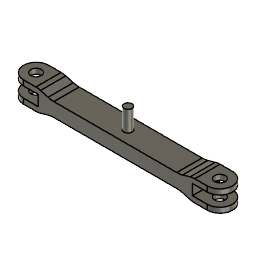
BARRA_SERVO (Autodesk Fusion 360 design; units mm, degrees)
Autodesk Fusion 360 part; units mm, degrees
sketch "Boceto1" plane through (0, 0, 0) normal (0, 0, 1) x (1, 0, 0)
  line L0 (-43.4775, 6) -> (43.4775, 6)
  circle A0 centre (0, 0) radius 1.95
  line L1 (-36.4775, 6) -> (-36.4775, -6)
  line L2 (36.4775, 6) -> (36.4775, -6)
  line L3 (-30.4775, 6) -> (-30.4775, -6)
  line L4 (30.4775, 6) -> (30.4775, -6)
  circle A1 centre (-43.4775, 0) radius 2 construction
  circle A2 centre (43.4775, 0) radius 2 construction
  line L5 (-43.4775, 0) -> (43.4775, 0) construction
  line L6 (-43.4868, -6) -> (43.4868, -6)
  arc A3 (-43.4775, 6) -> (-43.4868, -6) centre (-43.4775, 0) ccw
  arc A4 (43.4868, -6) -> (43.4775, 6) centre (43.4775, 0) ccw
  circle A5 centre (-43.4775, 0) radius 2.5
  circle A6 centre (43.4775, 0) radius 2.5
  line L7 (57, 0) -> (-57, 0) construction
  line L8 (0, -7.1894) -> (0, 7.1894) construction
  point P0 (0, -6)
  point P1 (0, 6)
  dimension "d8" = 3.9
  dimension "d9" = 86.955
  dimension "d16" = 6
  dimension "d17" = 6
  dimension "d18" = 86.9549
  dimension "d22" = 6
  dimension "d23" = 6
  dimension "d25" = 7
  dimension "d26" = 7
  dimension "d27" = 5
  dimension "d28" = 5
  constraint coincident A0.centre origin
  constraint coincident L0 L1.start
  constraint perpendicular L0 L1
  constraint coincident L0 L2.start
  constraint coincident L0 L3.start
  constraint perpendicular L0 L3
  constraint coincident L0 L4.start
  constraint coincident A1.centre L5.start
  constraint coincident A2.centre L5.end
  constraint perpendicular L2 L5
  constraint midpoint A0.centre L5
  constraint parallel L0 L6
  constraint tangent L0 A3
  constraint tangent L0 A4
  constraint coincident L1.end L6
  constraint coincident L3.end L6
  constraint coincident L4.end L6
  constraint coincident L2.end L6
  constraint concentric A1 A5
  constraint concentric A2 A6
  constraint midpoint L6 P0
  constraint midpoint L0 P1
  constraint midpoint L7 A0.centre
  constraint horizontal L7
  constraint coincident A1.centre L7
  constraint midpoint L8 A0.centre
  constraint perpendicular L7 L8
  constraint coincident P1 L8
  constraint coincident P0 L8
  measures "d8" diameter of A0
  measures "d9" distance of L0.start L0.end
  measures "d16" distance of L2 L4
  measures "d17" distance of L1 L3
  measures "d18" distance of A2.centre A1.centre
  measures "d22" distance of L5 L6
  measures "d23" distance of L0 L5
  measures "d25" distance of L2 A2.centre
  measures "d26" distance of L1 A1.centre
  measures "d27" diameter of A5
  measures "d28" diameter of A6
extrude "Extruir1" add sketch "Boceto1" along normal blind 10
sketch "Boceto2" plane through (0, -6, 0) normal (0, -1, 0) x (1, 0, 0)
  line L0 (-43.4868, 0) -> (43.4868, 0)
  line L1 (43.4868, 0) -> (43.4868, 10)
  line L2 (43.4868, 10) -> (-43.4868, 10)
  line L3 (-43.4868, 10) -> (-43.4868, 0)
  line L4 (-44.4258, 7.5) -> (-36.4775, 7.5)
  line L5 (-36.4775, 7.5) -> (-36.4775, 2.5)
  line L6 (-36.4775, 2.5) -> (-45, 2.5)
  line L7 (-43.4868, 0) -> (43.4868, 0)
  line L8 (-36.4775, 0) -> (-36.4775, 10) construction
  line L9 (-30.4775, 0) -> (-30.4775, 10) construction
  line L10 (-36.4775, 10) -> (-30.4775, 8.2795)
  line L11 (-36.4775, 0) -> (-30.4775, 1.7205)
  line L12 (0, 0) -> (0, 10) construction
  line L13 (0, 8.2795) -> (-30.4775, 8.2795)
  line L14 (0, 1.7205) -> (-30.4775, 1.7205)
  line L15 (36.4775, 2.5) -> (45, 2.5)
  line L16 (36.4775, 0) -> (36.4775, 10)
  line L17 (30.4775, 0) -> (30.4775, 10)
  line L18 (44.4258, 7.5) -> (36.4775, 7.5)
  line L19 (36.4775, 10) -> (30.4775, 8.2795)
  line L20 (36.4775, 0) -> (30.4775, 1.7205)
  line L21 (36.4775, 7.5) -> (36.4775, 2.5)
  line L22 (0, 8.2795) -> (30.4775, 8.2795)
  line L23 (0, 1.7205) -> (30.4775, 1.7205)
  point P0 (-36.4775, 0)
  point P1 (-30.4775, 0)
  point P2 (30.4775, 0)
  point P3 (36.4775, 0)
  dimension "d32" = 2.5
  dimension "d33" = 2.5
  dimension "d34" = 164
  dimension "d35" = 164
  constraint perpendicular L3 L4
  constraint perpendicular L4 L5
  constraint perpendicular L3 L6
  constraint coincident L7 P0
  constraint coincident L7 P1
  constraint coincident P0 L8.start
  constraint coincident L2 L8.end
  constraint perpendicular L2 L8
  constraint coincident P1 L9.start
  constraint coincident L2 L9.end
  constraint perpendicular L2 L9
  constraint collinear L5 L8
  constraint coincident L9 L10.end
  constraint coincident L9 L11.end
  constraint coincident L12.start origin
  constraint coincident L2 L12.end
  constraint perpendicular L2 L12
  constraint coincident L12 L13.start
  constraint perpendicular L9 L13
  constraint coincident L12 L14.start
  constraint symmetric L4.start L12 L18.start
  constraint symmetric L4.end L12 L18.end
  constraint symmetric L5.end L12 L15.start
  constraint symmetric L6.end L12 L15.end
  constraint symmetric P0 L12 P3
  constraint symmetric P1 L12 P2
  constraint symmetric L8.end L12 L16.end
  constraint symmetric L9.end L12 L17.end
  constraint symmetric L10.end L12 L19.end
  constraint symmetric L11.end L12 L20.end
  constraint symmetric L12 L13.start L22.start
  constraint symmetric L12 L14.start L23.start
  measures "d32" distance of L2 L4
  measures "d33" distance of L6 L7
  measures "d34" angle of L2 L10
  measures "d35" angle of L7 L11
extrude "Extruir2" cut sketch "Boceto2" against normal blind 17 contours L0 L7 L11 L14 L17 L23 | L0 L7 L17 L20 | L2 L10 L13 L17 L22 | L2 L17 L19
extrude "Extruir3" cut sketch "Boceto2" against normal blind 20 contours L3 L4 L5 L6 | L1 L15 L16 L18 L21
sketch "Boceto4" plane through (-36.4775, 0, 0) normal (-1, 0, 0) x (0, -1, 0)
  line L0 (-6, 7.5) -> (-6, 2.5)
  line L1 (-6, 2.5) -> (6, 2.5)
  line L2 (6, 2.5) -> (6, 7.5)
  line L3 (6, 7.5) -> (-6, 7.5)
  line L4 (-6, 7.5) -> (6, 7.5)
  line L5 (-6, 2.5) -> (6, 2.5)
  line L6 (6, 10) -> (-6, 10)
  line L7 (6, 0) -> (-6, 0)
  dimension "d40" = 2.5
  dimension "d41" = 2.5
  constraint coincident L0.start L3.end
  constraint coincident L2.end L3.start
  constraint perpendicular L2 L5
  measures "d40" distance of L4 L6
  measures "d41" distance of L5 L7
extrude "Extruir4" cut sketch "Boceto4" along normal blind 16
sketch "Boceto5" plane through (36.4775, 0, 0) normal (1, 0, 0) x (0, 1, 0)
  line L0 (6, 2.5) -> (6, 7.5)
  line L1 (6, 7.5) -> (-6, 7.5)
  line L2 (-6, 7.5) -> (-6, 2.5)
  line L3 (-6, 2.5) -> (6, 2.5)
  line L4 (6, 7.5) -> (-6, 7.5)
  line L5 (-6, 2.5) -> (6, 2.5)
  constraint coincident L0.end L1.start
  constraint coincident L1.end L2.start
  constraint coincident L2.end L3.start
  constraint coincident L0.start L3.end
extrude "Extruir5" cut sketch "Boceto5" along normal blind 27
extrude "Extruir6" add sketch "Boceto1" along normal blind 18 contours A0
extrude "Extruir7" cut sketch "Boceto2" against normal blind 20 contours L0 L7 L11 L14 L17 L23
fillet "Empalme1" radius 10 2 edges at (30.4775, 0, 8.2795) (-30.4775, 0, 8.2795)
fillet "Empalme2" radius 8 2 edges at (-36.4775, 0, 10) (36.4775, 0, 10)
fillet "Empalme3" radius 10 2 edges at (-30.4775, 0, 1.7205) (30.4775, 0, 1.7205)
fillet "Empalme4" radius 8 2 edges at (-36.4775, 0, 0) (36.4775, 0, 0)
sketch "Boceto6" plane through (0, -6, 0) normal (0, -1, 0) x (1, 0, 0)
  arc A0 (35.3967, 0.3099) -> (37.6018, 0) centre (37.6018, 8) ccw
  line L0 (37.6018, 0) -> (43.4868, 0)
  line L1 (43.4868, 0) -> (43.4868, 2.5)
  line L2 (43.4868, 2.5) -> (36.4775, 2.5)
  line L3 (36.4775, 2.5) -> (36.4775, 7.5)
  line L4 (36.4775, 7.5) -> (43.4868, 7.5)
  line L5 (43.4868, 7.5) -> (43.4868, 10)
  line L6 (43.4868, 10) -> (37.6018, 10)
  arc A1 (37.6018, 10) -> (35.3967, 9.6901) centre (37.6018, 2) ccw
  line L7 (35.3967, 9.6901) -> (31.8285, 8.6669)
  arc A2 (29.0721, 8.2795) -> (31.8285, 8.6669) centre (29.0721, 18.2795) ccw
  line L8 (29.0721, 8.2795) -> (-29.0721, 8.2795)
  arc A3 (-31.8285, 8.6669) -> (-29.0721, 8.2795) centre (-29.0721, 18.2795) ccw
  line L9 (-31.8285, 8.6669) -> (-35.3967, 9.6901)
  arc A4 (-35.3967, 9.6901) -> (-37.6018, 10) centre (-37.6018, 2) ccw
  line L10 (-37.6018, 10) -> (-43.4868, 10)
  line L11 (-43.4868, 10) -> (-43.4868, 7.5)
  line L12 (-43.4868, 7.5) -> (-36.4775, 7.5)
  line L13 (-36.4775, 7.5) -> (-36.4775, 2.5)
  line L14 (-36.4775, 2.5) -> (-43.4868, 2.5)
  line L15 (-43.4868, 2.5) -> (-43.4868, 0)
  line L16 (-43.4868, 0) -> (-37.6018, 0)
  arc A5 (-37.6018, 0) -> (-35.3967, 0.3099) centre (-37.6018, 8) ccw
  line L17 (-35.3967, 0.3099) -> (-31.8285, 1.3331)
  arc A6 (-29.0721, 1.7205) -> (-31.8285, 1.3331) centre (-29.0721, -8.2795) ccw
  line L18 (-29.0721, 1.7205) -> (29.0721, 1.7205)
  arc A7 (31.8285, 1.3331) -> (29.0721, 1.7205) centre (29.0721, -8.2795) ccw
  line L19 (31.8285, 1.3331) -> (35.3967, 0.3099)
  line L20 (-29.0721, 1.7205) -> (29.0721, 1.7205)
  line L21 (36.4775, 7.5) -> (43.4868, 7.5)
  line L22 (36.4775, 2.5) -> (36.4775, 7.5)
  arc A8 (31.8285, 1.3331) -> (29.0721, 1.7205) centre (29.0721, -8.2795) ccw
  line L23 (31.8285, 1.3331) -> (35.3967, 0.3099)
  arc A9 (35.3967, 0.3099) -> (37.6018, 0) centre (37.6018, 8) ccw
  line L24 (37.6018, 0) -> (43.4868, 0)
  line L25 (43.4868, 0) -> (43.4868, 2.5)
  line L26 (43.4868, 2.5) -> (36.4775, 2.5)
  line L27 (43.4868, 7.5) -> (43.4868, 10)
  line L28 (37.6018, 10) -> (43.4868, 10)
  arc A10 (37.6018, 10) -> (35.3967, 9.6901) centre (37.6018, 2) ccw
  line L29 (35.3967, 9.6901) -> (31.8285, 8.6669)
  arc A11 (29.0721, 8.2795) -> (31.8285, 8.6669) centre (29.0721, 18.2795) ccw
  line L30 (29.0721, 8.2795) -> (-29.0721, 8.2795)
  arc A12 (-31.8285, 8.6669) -> (-29.0721, 8.2795) centre (-29.0721, 18.2795) ccw
  line L31 (-31.8285, 8.6669) -> (-35.3967, 9.6901)
  arc A13 (-35.3967, 9.6901) -> (-37.6018, 10) centre (-37.6018, 2) ccw
  line L32 (-43.4868, 10) -> (-37.6018, 10)
  line L33 (-43.4868, 7.5) -> (-43.4868, 10)
  line L34 (-43.4868, 7.5) -> (-36.4775, 7.5)
  line L35 (-36.4775, 2.5) -> (-43.4868, 2.5)
  line L36 (-36.4775, 7.5) -> (-36.4775, 2.5)
  line L37 (-43.4868, 0) -> (-43.4868, 2.5)
  line L38 (-43.4868, 0) -> (-37.6018, 0)
  arc A14 (-37.6018, 0) -> (-35.3967, 0.3099) centre (-37.6018, 8) ccw
  line L39 (-35.3967, 0.3099) -> (-31.8285, 1.3331)
  arc A15 (-29.0721, 1.7205) -> (-31.8285, 1.3331) centre (-29.0721, -8.2795) ccw
